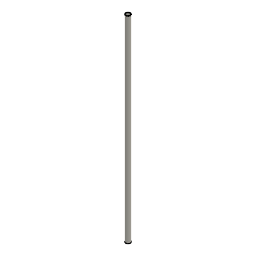
Soporte (Autodesk Fusion 360 design; units mm, degrees)
part number: 2025-09-05-15-57-09-061
Autodesk Fusion 360 part; units mm, degrees
sketch "Boceto1" plane through (0, 0, 0) normal (0, 0, 1) x (1, 0, 0)
  circle A0 centre (0, 0) radius 10.58
  dimension "d1" = 21.16
  constraint coincident A0.centre origin
  measures "d1" diameter of A0
extrude "Extruir1" add sketch "Boceto1" along normal blind 865.7
sketch "Boceto2" plane through (0, 0, 865.7) normal (0, 0, 1) x (-1, 0, 0)
  circle A0 centre (0, 0) radius 10.58
  circle A1 centre (0, 0) radius 8.75
  dimension "d4" = 17.5
  constraint coincident A0.centre A1.centre
  measures "d4" diameter of A1
extrude "Extruir2" cut sketch "Boceto2" against normal blind 870 contours A1
